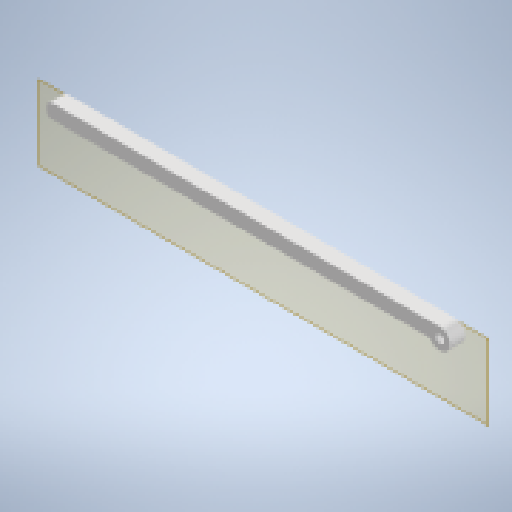
# Autodesk Inventor part: flip-stand-bottom
Saved by Autodesk Inventor 2023 (Build 270158030, 158C)
## iProperties
Created: 2023-04-28
Part Number: flip-stand-bottom
Material: Generic
Document SubType Name: Modeling
Designer: Imogen Heard
Density: 1 g/cm^3
Appearance: Default
Author: Imogen Heard
Autodesk Inventor part; units mm, degrees
ref_plane "YZ Plane" through (0, 0, 0) normal (1, 0, 0) x (0, 1, 0)
ref_plane "XZ Plane" through (0, 0, 0) normal (0, 1, 0) x (-1, 0, 0)
ref_plane "XY Plane" through (0, 0, 0) normal (0, 0, 1) x (1, 0, 0)
ref_plane "Work Plane1" through (0, 0, 0) normal (0, 0, 1) x (1, 0, 0)
sketch "Sketch1" plane through (0, 0, 0) normal (0, 0, 1) x (1, 0, 0)
  circle A0 centre (77.9, 1) radius 0.8 projected
  line L0 (79.585, 1.6) -> (78.4292, 1.6) construction
  line L1 (2.9, 3) -> (77.9, 3)
  arc A1 (2.9, 3) -> (2.9, 0.2) centre (2.9, 1.6) ccw
  arc A2 (76.4, -0.3229) -> (77.9, 3) centre (77.9, 1) ccw
  line L2 (75.0516, 0.2) -> (2.9, 0.2)
  arc A3 (76.4, -0.3229) -> (75.0516, 0.2) centre (75.0516, -1.8) ccw
  point P0 (0, 0)
  point P1 (41.1836, 1.6)
  point P2 (74.7858, 0.2)
  dimension "d1" = 4
  dimension "d2" = 2.8
  dimension "d4" = 2
  dimension "d5" = 75
  dimension "d6" = 1.5
  constraints: 7 end point, 6 point on circle, 3 centre point, 3 point on line, 3 tangent, 2 horizontal, 1 parallel, 1 vertical alignment, 3 other
  measures "d1" diameter of A2
  measures "d2" distance between parallel lines of L1 L2
  measures "d4" radius of A3
  measures "d5" horizontal distance of point (77.9, 1) A1.centre
  measures "d6" horizontal distance of point (77.9, 1) A2.start
extrude "Extrusion1" add sketch "Sketch1" along normal blind 3
body "Solid1"
